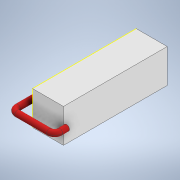
# Autodesk Inventor part: lipol 150mAH
Saved by Autodesk Inventor 2022.3 (Build 263350000, 350)
## iProperties
Created: 2022-12-13
Part Number: lipol 150mAH
Material: Generic
Document SubType Name: Modeling
Designer: komputer
Density: 1 g/cm^3
Appearance: Default
Author: komputer
Autodesk Inventor part; units mm, degrees
ref_plane "YZ Plane" through (0, 0, 0) normal (1, 0, 0) x (0, 1, 0)
ref_plane "XZ Plane" through (0, 0, 0) normal (0, 1, 0) x (-1, 0, 0)
ref_plane "XY Plane" through (0, 0, 0) normal (0, 0, 1) x (1, 0, 0)
sketch "Sketch1" plane through (0, 0, 0) normal (0, 0, 1) x (1, 0, 0)
  line L0 (-2.9135, 2.0782) -> (9.0865, 2.0782)
  line L1 (9.0865, 2.0782) -> (9.0865, -10.9218)
  line L2 (9.0865, -10.9218) -> (-2.9135, -10.9218)
  line L3 (-2.9135, -10.9218) -> (-2.9135, 2.0782)
  point P0 (0, 0)
  dimension "d0" = 12
  dimension "d1" = 13
  constraints: 8 end point, 2 parallel, 1 horizontal, 1 perpendicular
  measures "d0" distance of L1.end L2.end
  measures "d1" distance of L0.end L1.end
extrude "Extrusion1" add sketch "Sketch1" along normal blind 40
sketch "Sketch2" plane through (-2.9135, -10.9218, 0) normal (-1, 0, 0) x (0, 0, 1)
  line L0 (0, 13) -> (0, 0) projected
  line L1 (0, 0) -> (40, 0) projected
  line L2 (40, 13) -> (40, 0) projected
  line L3 (0, 13) -> (40, 13) projected
  line L4 (40, 0) -> (40, 13) projected
  circle A0 centre (34.2104, 6.5) radius 1.1119
  point P0 (0, 10.9218)
  constraints: 1 centre point, 1 coincident
sketch "Sketch3" plane through (0, 0, 40) normal (0, 0, 1) x (1, 0, 0)
  line L0 (-2.9135, -10.9218) -> (9.0865, -10.9218) projected
  line L1 (9.0865, -10.9218) -> (9.0865, 2.0782) projected
  line L2 (9.0865, 2.0782) -> (-2.9135, 2.0782) projected
  line L3 (-2.9135, 2.0782) -> (-2.9135, -10.9218) projected
  line L4 (9.0865, -10.9218) -> (9.0865, 2.0782) projected
  line L5 (9.0865, -4.4218) -> (10.3126, -4.4218)
  circle A0 centre (10.3126, -4.4218) radius 1.112
  point P0 (0, 0)
  dimension "d4" = 2.224
  constraints: 2 end point, 1 centre point, 1 coincident, 1 horizontal, 1 midpoint
  measures "d4" diameter of A0
sketch3d "3D Sketch1"
  line L0 (10.3126, -4.4218, 40) -> (10.3552, -4.4218, 42.6616)
  arc A0 (10.3552, -4.4218, 42.6616) -> (8.3554, -4.4218, 44.6936) centre (8.3554, -4.4218, 42.6936) ccw
  line L1 (8.3554, -4.4218, 44.6936) -> (-3.9098, -4.4218, 44.6936)
  arc A1 (-3.9098, -4.4218, 44.6936) -> (-5.9098, -4.4218, 42.6936) centre (-3.9098, -4.4218, 42.6936) ccw
  line L2 (-5.9098, -4.4218, 42.6936) -> (-5.9098, -4.4218, 36.2104)
  arc A2 (-5.9098, -4.4218, 36.2104) -> (-3.9098, -4.4218, 34.2104) centre (-3.9098, -4.4218, 36.2104) ccw
  line L3 (-3.9098, -4.4218, 34.2104) -> (-2.9135, -4.4218, 34.2104)
  dimension "d5" = 2
  dimension "d6" = 2
  dimension "d7" = 2
sweep "Sweep1" add profiles "Sketch3" path "3D Sketch1" contours A0
equation "\"d6\" = d5"
equation "\"d7\" = d5"
body "Solid1"
